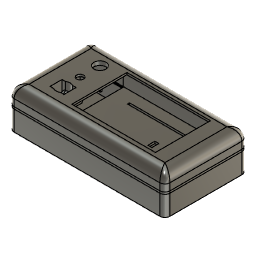
Case (Autodesk Fusion 360 design; units mm, degrees)
Autodesk Fusion 360 part; units mm, degrees
sketch "Base" plane through (0, 0, 0) normal (0, 0, 1) x (1, 0, 0)
  line L0 (1.2621, 68) -> (1.2621, 5)
  line L1 (1.2621, 5) -> (107, 5)
  line L2 (107, 5) -> (107, 68)
  line L3 (107, 68) -> (1.2621, 68)
  line L4 (-38.7379, 72.5) -> (-38.7379, 0.5)
  line L5 (-33.7379, -4.5) -> (112, -4.5)
  line L6 (117, 0.5) -> (117, 72.5)
  line L7 (112, 77.5) -> (-33.7379, 77.5)
  arc A0 (-33.7379, 77.5) -> (-38.7379, 72.5) centre (-33.7379, 72.5) ccw
  arc A1 (117, 72.5) -> (112, 77.5) centre (112, 72.5) ccw
  arc A2 (112, -4.5) -> (117, 0.5) centre (112, 0.5) ccw
  arc A3 (-38.7379, 0.5) -> (-33.7379, -4.5) centre (-33.7379, 0.5) ccw
  line L8 (39.1311, 77.5) -> (39.1311, -4.5)
  line L9 (-38.7379, 36.5) -> (117, 36.5)
  point P0 (-33.7379, 57.5)
  point P1 (-33.7379, 15.5)
  point P2 (112, 57.5)
  point P3 (112, 15.5)
  dimension "d4" = 9.5
  dimension "d5" = 10
  dimension "d7" = 5
  dimension "d8" = 40
  dimension "d72" = 9.5
  dimension "d73" = 63
  dimension "d74" = 105.7379
  dimension "d75" = 20
  dimension "d76" = 5
  constraint tangent L4 A0
  constraint tangent L7 A0
  constraint tangent L6 A1
  constraint tangent L7 A1
  constraint equal A0 A1
  constraint tangent L5 A2
  constraint tangent L6 A2
  constraint equal A0 A2
  constraint tangent L4 A3
  constraint tangent L5 A3
  constraint equal A0 A3
  constraint midpoint L7 L8.start
  constraint midpoint L5 L8.end
  constraint perpendicular L5 L8
  constraint midpoint L4 L9.start
  constraint midpoint L6 L9.end
  constraint symmetric L9 P0 P1
  constraint symmetric L8 P0 P2
  constraint symmetric L8 P1 P3
  measures "d4" distance of L1 L5
  measures "d5" distance of L2 L6
  measures "d7" radius of A0
  measures "d8" distance of L0 L4
  measures "d72" distance of L3 L7
  measures "d73" distance of L1 L3
  measures "d74" distance of L0 L2
  measures "d75" distance of L7 P0
  measures "d76" distance of L4 P0
extrude "Extrude1" add sketch "Base" along normal blind 20 makes body 1
sketch "Battery Inset" plane through (0, 0, 20) normal (0, 0, 1) x (-1, 0, 0)
  arc A0 (38.7379, -0.5) -> (33.7379, 4.5) centre (33.7379, -0.5) ccw
  line L0 (33.7379, 4.5) -> (-112, 4.5)
  arc A1 (-112, 4.5) -> (-117, -0.5) centre (-112, -0.5) ccw
  line L1 (-117, -0.5) -> (-117, -72.5)
  arc A2 (-117, -72.5) -> (-112, -77.5) centre (-112, -72.5) ccw
  line L2 (-112, -77.5) -> (33.7379, -77.5)
  arc A3 (33.7379, -77.5) -> (38.7379, -72.5) centre (33.7379, -72.5) ccw
  line L3 (38.7379, -72.5) -> (38.7379, -0.5)
  line L4 (-6.5, -68) -> (-107, -68)
  line L5 (-107, -68) -> (-107, -5)
  line L6 (-107, -5) -> (-6.5, -5)
  line L7 (-6.5, -5) -> (-6.5, -68)
  line L8 (-6.5, -36.5) -> (-107, -36.5) construction
  line L9 (38.7379, -36.5) -> (-117, -36.5) construction
  line L10 (28.7379, -68) -> (-107, -68)
  line L11 (-107, -68) -> (-107, -5)
  line L12 (-107, -5) -> (28.7379, -5)
  line L13 (28.7379, -5) -> (28.7379, -68)
  line L14 (-1.2621, -5) -> (-107, -5)
  line L15 (-107, -5) -> (-107, -68)
  line L16 (-107, -68) -> (-1.2621, -68)
  line L17 (38.7379, -72.5) -> (38.7379, -0.5)
  line L18 (-6.5, -68) -> (-3.5, -68)
  line L19 (-3.5, -68) -> (-3.5, -5)
  line L20 (-3.5, -5) -> (-6.5, -5)
  line L21 (-6.5, -5) -> (-6.5, -68)
  line L22 (-3.5, -12) -> (-6.5, -12)
  line L23 (-3.5, -30) -> (-6.5, -30)
  line L24 (-18.5, -44) -> (-22.5, -44)
  line L25 (-22.5, -44) -> (-22.5, -29)
  line L26 (-22.5, -29) -> (-18.5, -29)
  line L27 (-18.5, -29) -> (-18.5, -44)
  line L28 (-18.5, -36.5) -> (-22.5, -36.5) construction
  line L29 (-20.5, -44) -> (-20.5, -29) construction
  dimension "d168" = 63
  dimension "d169" = 100.5
  dimension "d170" = 10
  dimension "d171" = 3
  dimension "d174" = 15
  dimension "d175" = 4
  dimension "d176" = 14
  dimension "d188" = 7
  dimension "d189" = 25
  constraint horizontal L4
  constraint vertical L5
  constraint horizontal L6
  constraint vertical L7
  constraint midpoint L7 L8.start
  constraint midpoint L5 L8.end
  constraint collinear L8 L9
  constraint horizontal L10
  constraint vertical L11
  constraint horizontal L12
  constraint vertical L13
  constraint collinear L12 L14
  constraint collinear L11 L15
  constraint collinear L10 L16
  constraint horizontal L18
  constraint vertical L19
  constraint horizontal L20
  constraint vertical L21
  constraint collinear L6 L20
  constraint coincident L19 L22.start
  constraint coincident L7 L22.end
  constraint perpendicular L7 L22
  constraint coincident L19 L23.start
  constraint coincident L7 L23.end
  constraint perpendicular L7 L23
  constraint horizontal L24
  constraint vertical L25
  constraint horizontal L26
  constraint vertical L27
  constraint midpoint L27 L28.start
  constraint midpoint L25 L28.end
  constraint collinear L8 L28
  constraint midpoint L24 L29.start
  constraint midpoint L26 L29.end
  constraint collinear L5 L11
  measures "d168" distance of L4 L6
  measures "d169" distance of L5 L7
  measures "d170" distance of L13 L17
  measures "d171" distance of L7 L19
  measures "d174" distance of L24 L26
  measures "d175" distance of L25 L27
  measures "d176" distance of L7 L29
  measures "d188" distance of L20 L22
  measures "d189" distance of L20 L23
extrude "Extrude2" cut sketch "Battery Inset" against normal blind 17 contours L4 L5 L6 L7 L10 L11 L12 L14 L15 L16 L21 | L7 L19 L21 L22 L23 | L10 L12 L13 L14 L16 L19 | L24 L25 L26 L27 bodies 1
extrude "Extrude17" cut sketch "Battery Inset" against normal through all contours L24 L25 L26 L27 bodies 1
fillet "Fillet3" radius 0.5 12 edges at (56.75, 68, 20) (107, 36.5, 20) (56.75, 5, 20) (6.5, 49, 20) (5, 30, 20) (3.5, 49, 20) (-12.6189, 68, 20) (-28.7379, 36.5, 20) (-12.6189, 5, 20) (3.5, 8.5, 20) (6.5, 8.5, 20) (5, 12, 20) on bodies 1
sketch "Top Base" plane through (0, 0, 20) normal (0, 0, 1) x (-1, 0, 0)
  arc A0 (38.7379, -0.5) -> (33.7379, 4.5) centre (33.7379, -0.5) ccw
  line L0 (33.7379, 4.5) -> (-112, 4.5)
  arc A1 (-112, 4.5) -> (-117, -0.5) centre (-112, -0.5) ccw
  line L1 (-117, -0.5) -> (-117, -72.5)
  arc A2 (-117, -72.5) -> (-112, -77.5) centre (-112, -72.5) ccw
  line L2 (-112, -77.5) -> (33.7379, -77.5)
  arc A3 (33.7379, -77.5) -> (38.7379, -72.5) centre (33.7379, -72.5) ccw
  line L3 (38.7379, -72.5) -> (38.7379, -0.5)
  line L4 (29.2379, -68.5) -> (-4, -68.5)
  line L5 (-4, -68.5) -> (-4, -4.5)
  line L6 (-4, -4.5) -> (29.2379, -4.5)
  line L7 (29.2379, -4.5) -> (29.2379, -68.5)
  line L8 (-100.5103, -56.4999) -> (-100.5103, -10.4999)
  line L9 (-96.5103, -6.4999) -> (-20.5103, -6.4999)
  line L10 (-20.5103, -54.4999) -> (-92.5415, -54.4999)
  line L11 (-96.5103, -54.4999) -> (-96.5103, -10.4999)
  line L12 (-96.5103, -8.4999) -> (-20.5103, -8.4999)
  line L13 (-66.5103, -35.9999) -> (-70.5103, -35.9999)
  line L14 (-70.5103, -35.9999) -> (-70.5103, -28.9999)
  line L15 (-70.5103, -28.9999) -> (-66.5103, -28.9999)
  line L16 (-66.5103, -28.9999) -> (-66.5103, -35.9999)
  circle A4 centre (-8.5103, -14.4999) radius 5
  line L17 (-20.5103, -6.4999) -> (-20.5103, -8.4999)
  line L18 (-20.5103, -54.4999) -> (-20.5103, -56.4999)
  line L19 (-96.5103, -6.4999) -> (-96.5103, -8.4999)
  line L20 (-96.5103, -10.4999) -> (-100.5103, -10.4999)
  line L21 (-92.5415, -54.4999) -> (-92.5415, -56.4999)
  line L22 (-96.5103, -56.4999) -> (-96.5103, -54.4999)
  line L23 (-20.5103, -56.4999) -> (-92.5415, -56.4999)
  line L24 (-96.5103, -56.4999) -> (-100.5103, -56.4999)
  line L25 (-6, -4.5) -> (-6, -11.5)
  line L26 (-6, -11.5) -> (-4, -11.5)
  line L27 (-4, -11.5) -> (-4, -4.5)
  line L28 (-4, -4.5) -> (29.2379, -4.5)
  line L29 (29.2379, -4.5) -> (29.2379, -68.5)
  line L30 (29.2379, -68.5) -> (-4, -68.5)
  line L31 (-4, -68.5) -> (-4, -30.5)
  line L32 (-4, -30.5) -> (-6, -30.5)
  line L33 (-6, -30.5) -> (-6, -68.5)
  line L34 (-6, -68.5) -> (-107.5, -68.5)
  line L35 (-107.5, -68.5) -> (-107.5, -4.5)
  line L36 (-107.5, -4.5) -> (-6, -4.5)
  dimension "d32" = 50
  dimension "d33" = 2
  dimension "d34" = 2
  dimension "d35" = 4
  dimension "d36" = 80
  dimension "d37" = 34
  dimension "d38" = 4
  dimension "d39" = 7
  dimension "d40" = 29.5
  dimension "d41" = 10
  dimension "d42" = 92
  dimension "d43" = 8
  constraint horizontal L4
  constraint vertical L5
  constraint horizontal L6
  constraint vertical L7
  constraint horizontal L23
  constraint vertical L8
  constraint horizontal L9
  constraint vertical L17
  constraint horizontal L10
  constraint vertical L11
  constraint horizontal L12
  constraint horizontal L13
  constraint vertical L14
  constraint horizontal L15
  constraint vertical L16
  constraint collinear L17 L18
  constraint vertical L19
  constraint horizontal L20
  constraint vertical L21
  constraint vertical L22
  constraint collinear L23 L24
  constraint collinear L7 L29
  constraint collinear L4 L30
  constraint collinear L6 L28
  constraint collinear L5 L27
  measures "d32" distance of L9 L23
  measures "d33" distance of L10 L23
  measures "d34" distance of L9 L12
  measures "d35" distance of L8 L11
  measures "d36" distance of L8 L17
  measures "d37" distance of L8 L16
  measures "d38" distance of L14 L16
  measures "d39" distance of L13 L15
  measures "d40" distance of L9 L13
  measures "d41" diameter of A4
  measures "d42" distance of L8 A4.centre
  measures "d43" distance of L9 A4.centre
extrude "Extrude5" add sketch "Top Base" along normal blind 2 separate body contours A0 L0 A1 L1 A2 L2 A3 L3 | L5 A4 L25 L32 L33 L34 L35 L36 | L5 A4 L26 makes body 2
sketch "Top" plane through (0, 0, 22) normal (0, 0, 1) x (-1, 0, 0)
  line L0 (38.7379, -72.5) -> (38.7379, -0.5)
  arc A0 (38.7379, -0.5) -> (33.7379, 4.5) centre (33.7379, -0.5) ccw
  line L1 (33.7379, 4.5) -> (-112, 4.5)
  arc A1 (-112, 4.5) -> (-117, -0.5) centre (-112, -0.5) ccw
  line L2 (-117, -0.5) -> (-117, -72.5)
  arc A2 (-117, -72.5) -> (-112, -77.5) centre (-112, -72.5) ccw
  line L3 (-112, -77.5) -> (33.7379, -77.5)
  arc A3 (33.7379, -77.5) -> (38.7379, -72.5) centre (33.7379, -72.5) ccw
  line L4 (-3.4004, -67.4999) -> (-105.5103, -67.4999)
  line L5 (-105.5103, -67.4999) -> (-105.5103, -4.4999)
  line L6 (-105.5103, -4.4999) -> (-3.4004, -4.4999)
  line L7 (-3.4004, -4.4999) -> (-3.4004, -67.4999)
  line L8 (28.7379, -67.5) -> (-3.4004, -67.5)
  line L9 (-3.4004, -67.5) -> (-3.4004, -5.5)
  line L10 (-3.4004, -5.5) -> (28.7379, -5.5)
  line L11 (28.7379, -5.5) -> (28.7379, -67.5)
  line L12 (-96.5103, -8.4999) -> (-96.5103, -6.4999)
  line L13 (-100.5103, -10.4999) -> (-96.5103, -10.4999)
  line L14 (-20.5103, -56.4999) -> (-92.5415, -56.4999)
  line L15 (-92.5415, -56.4999) -> (-92.5415, -54.4999)
  line L16 (-96.5103, -8.4999) -> (-20.5103, -8.4999)
  line L17 (-96.5103, -54.4999) -> (-96.5103, -10.4999)
  line L18 (-4, -68.5) -> (-4, -16.658)
  line L19 (-93.5103, -67.4999) -> (-93.5103, -4.4999)
  dimension "d54" = 10
  dimension "d55" = 10
  dimension "d56" = 10
  dimension "d77" = 4
  dimension "d78" = 9
  dimension "d192" = 12
  constraint horizontal L4
  constraint vertical L5
  constraint horizontal L6
  constraint vertical L7
  constraint horizontal L8
  constraint vertical L9
  constraint horizontal L10
  constraint vertical L11
  constraint collinear L7 L9
  constraint coincident L4 L19.start
  constraint coincident L6 L19.end
  constraint perpendicular L6 L19
  measures "d54" distance of L3 L8
  measures "d55" distance of L1 L10
  measures "d56" distance of L0 L11
  measures "d77" distance of L6 L16
  measures "d78" distance of L5 L17
  measures "d192" distance of L5 L19
extrude "Extrude6" add sketch "Top" along normal blind 17 separate body contours L0 A0 L1 A1 L2 A2 L3 A3 | L4 L6 L7 L9 L19 | L4 L5 L6 L19 | L7 L8 L9 L10 L11 makes body 3
extrude "Extrude7" cut sketch "Top" along normal blind 15 contours L4 L6 L7 L9 L19 | L4 L5 L6 L19 bodies 3
extrude "Extrude8" cut sketch "Top" along normal blind 13 contours L7 L8 L9 L10 L11 bodies 3
extrude "Extrude19" cut sketch "Top" along normal blind 15.5 contours L4 L5 L6 L19 bodies 3
sketch "Screen Cutout" plane through (0, 0, 39) normal (0, 0, 1) x (-1, 0, 0)
  arc A0 (33.7379, -77.5) -> (38.7379, -72.5) centre (33.7379, -72.5) ccw
  line L0 (38.7379, -72.5) -> (38.7379, -0.5)
  arc A1 (38.7379, -0.5) -> (33.7379, 4.5) centre (33.7379, -0.5) ccw
  line L1 (33.7379, 4.5) -> (-112, 4.5)
  arc A2 (-112, 4.5) -> (-117, -0.5) centre (-112, -0.5) ccw
  line L2 (-117, -0.5) -> (-117, -72.5)
  arc A3 (-117, -72.5) -> (-112, -77.5) centre (-112, -72.5) ccw
  line L3 (-112, -77.5) -> (33.7379, -77.5)
  line L4 (-10.0103, -64.4999) -> (-93.5103, -64.4999)
  line L5 (-93.5103, -64.4999) -> (-93.5103, -9.4999)
  line L6 (-93.5103, -9.4999) -> (-10.0103, -9.4999)
  line L7 (-10.0103, -9.4999) -> (-10.0103, -64.4999)
  dimension "d59" = 83.5
  dimension "d60" = 55
  constraint horizontal L4
  constraint vertical L5
  constraint horizontal L6
  constraint vertical L7
  measures "d59" distance of L5 L7
  measures "d60" distance of L4 L6
extrude "Extrude9" cut sketch "Screen Cutout" against normal through all contours L4 L5 L6 L7 bodies 3
fillet "Fillet4" radius 10 8 edges at (117, 36.5, 39) (115.5355, 76.0355, 39) (39.1311, 77.5, 39) (-37.2734, 76.0355, 39) (-38.7379, 36.5, 39) (-37.2734, -3.0355, 39) (39.1311, -4.5, 39) (115.5355, -3.0355, 39) on bodies 3
hole "Hole2" at (-33.7379, 15.5, 0) at (-33.7379, 57.5, 0) at (112, 15.5, 0) at (112, 57.5, 0) direction (0, 0, 1) diameter 3.5 depth 30 tip angle 180 countersink diameter 7 countersink angle 90 bodies 1 2 3
ref_plane "WorkPlane1" through (39.1311, 36.5, 24) normal (0, 0, -1) x (1, 0, 0)
sketch "Insets" plane through (39.1311, 36, 24) normal (0, 0, -1) x (1, 0, 0)
  line L0 (77.8689, 35.5) -> (77.8689, -36.5)
  line L1 (67.8689, 31) -> (67.8689, -32)
  line L2 (-77.8689, -0.5) -> (77.8689, -0.5)
  line L3 (66.3792, -31.4999) -> (66.3792, 31.5001)
  line L4 (-77.8689, -36.5) -> (-77.8689, 35.5)
  line L5 (-67.8689, 30.5) -> (-67.8689, -31.5)
  line L6 (72.8689, -41.5) -> (-72.8689, -41.5)
  circle A0 centre (-72.8689, -21.5) radius 2.3
  circle A1 centre (72.8689, -21.5) radius 2.3
  circle A2 centre (-72.8689, 20.5) radius 2.3
  circle A3 centre (72.8689, 20.5) radius 2.3
  point P0 (-72.8689, -21.5)
  point P1 (72.8689, -21.5)
  point P2 (-72.8689, 21)
  point P3 (72.8689, 21)
  dimension "d193" = 4.6
  constraint coincident P0 A0.centre
  constraint coincident P1 A1.centre
  constraint equal A0 A1
  constraint symmetric L2 A0 A2
  constraint symmetric L2 A1 A3
  measures "d193" diameter of A0
extrude "Thread inserts cut" cut sketch "Insets" against normal blind 7.5 from surface at 2 bodies 3
chamfer "Chamfer6" distance 1 angle 45 4 edges at (109.8556, 56.6683, 22) (109.8556, 14.6683, 22) (-35.8823, 14.6683, 22) (-35.8823, 56.6683, 22) on bodies 3
sketch "Buttons" plane through (0, 0, 39) normal (0, 0, 1) x (-1, 0, 0)
  line L0 (-10.0103, -9.4999) -> (-10.0103, -64.4999)
  line L1 (-10.0103, -64.4999) -> (-93.5103, -64.4999)
  line L2 (-93.5103, -64.4999) -> (-93.5103, -9.4999)
  line L3 (-93.5103, -9.4999) -> (-10.0103, -9.4999)
  line L4 (-107, -5.5) -> (-107, -67.5)
  line L5 (-107, -67.5) -> (28.7379, -67.5)
  line L6 (28.7379, -67.5) -> (28.7379, -5.5)
  line L7 (28.7379, -5.5) -> (-107, -5.5)
  circle A0 centre (9.3638, -56.9428) radius 6
  circle A1 centre (9.3638, -37.1549) radius 3.5
  line L8 (18.3638, -28.1549) -> (18.3638, -46.1549)
  line L9 (18.3638, -46.1549) -> (-3.6362, -46.1549)
  line L10 (-3.6362, -46.1549) -> (-3.6362, -28.1549)
  line L11 (-3.6362, -28.1549) -> (18.3638, -28.1549)
  line L12 (19.25, -47.7455) -> (-1.9181, -47.7455)
  line L13 (-1.9181, -47.7455) -> (-1.9181, -12.0036)
  line L14 (-1.9181, -12.0036) -> (19.25, -12.0036)
  line L15 (19.25, -12.0036) -> (19.25, -47.7455)
  line L16 (16.3638, -26.0524) -> (2.3638, -26.0524)
  line L17 (2.3638, -26.0524) -> (2.3638, -14.0524)
  line L18 (2.3638, -14.0524) -> (16.3638, -14.0524)
  line L19 (16.3638, -14.0524) -> (16.3638, -26.0524)
  line L20 (9.3638, -26.0524) -> (9.3638, -14.0524) construction
  line L21 (16.3638, -20.0524) -> (2.3638, -20.0524) construction
  circle A2 centre (9.3638, -20.0524) radius 7
  line L22 (-10.0103, -64.4999) -> (28.7379, -64.4999) construction
  line L23 (9.3638, -64.4999) -> (9.3638, -5.5) construction
  line L24 (14.3638, -26.0524) -> (14.3638, -14.0524)
  line L25 (4.3638, -26.0524) -> (4.3638, -14.0524)
  line L26 (10.6138, -29.6049) -> (8.1138, -29.6049)
  line L27 (8.1138, -29.6049) -> (8.1138, -28.4049)
  line L28 (8.1138, -28.4049) -> (10.6138, -28.4049)
  line L29 (10.6138, -28.4049) -> (10.6138, -29.6049)
  line L30 (9.3638, -29.6049) -> (9.3638, -28.4049)
  circle A3 centre (9.3638, -37.1549) radius 6
  dimension "d122" = 12
  dimension "d124" = 7
  dimension "d125" = 18
  dimension "d126" = 22
  dimension "d127" = 9
  dimension "d128" = 9
  dimension "d145" = 14
  dimension "d146" = 12
  dimension "d147" = 14
  dimension "d152" = 2
  dimension "d153" = 2
  dimension "d198" = 2.5
  dimension "d199" = 1.2
  dimension "d200" = 8.75
  dimension "d204" = 12
  constraint horizontal L12
  constraint vertical L13
  constraint horizontal L14
  constraint vertical L15
  constraint horizontal L16
  constraint vertical L17
  constraint horizontal L18
  constraint vertical L19
  constraint midpoint L16 L20.start
  constraint midpoint L18 L20.end
  constraint midpoint L19 L21.start
  constraint midpoint L17 L21.end
  constraint midpoint L21 A2.centre
  constraint coincident L0.end L1.start
  constraint coincident L6 L22.end
  constraint perpendicular L6 L22
  constraint midpoint L22 L23.start
  constraint coincident L7 L23.end
  constraint perpendicular L7 L23
  constraint coincident A0.centre L23
  constraint coincident A2.centre L23
  constraint coincident A1.centre L23
  constraint coincident L16 L24.start
  constraint coincident L18 L24.end
  constraint perpendicular L18 L24
  constraint coincident L16 L25.start
  constraint coincident L18 L25.end
  constraint perpendicular L18 L25
  constraint horizontal L26
  constraint vertical L27
  constraint horizontal L28
  constraint vertical L29
  constraint midpoint L26 L30.start
  constraint midpoint L28 L30.end
  constraint collinear L23 L30
  constraint concentric A1 A3
  measures "d122" diameter of A0
  measures "d124" diameter of A1
  measures "d125" distance of L8.start L8.end
  measures "d126" distance of L8 L10
  measures "d127" distance of A1.centre L11
  measures "d128" distance of A1.centre L8
  measures "d145" distance of L17 L19
  measures "d146" distance of L16 L18
  measures "d147" diameter of A2
  measures "d152" distance of L17 L25
  measures "d153" distance of L19 L24
  measures "d198" distance of L26.start L26.end
  measures "d199" distance of L26.start L28.end
  measures "d200" distance of A1.centre L28
  measures "d204" diameter of A3
extrude "Extrude13" add sketch "Buttons" against normal blind 12 contours L8 L9 L11 L12 L13 L14 L15 | L16 L19 A2 L24 | L16 A2 L24 | L18 L19 A2 L24 | A2 L24 | L16 A2 | L16 L18 A2 L24 L25 | L18 A2 L24 | L16 A2 L25 | L18 A2 | L16 L17 A2 L25 | A2 L25 | L18 A2 L25 | L17 L18 A2 L25 bodies 3
extrude "Extrude11" cut sketch "Buttons" against normal through all contours A0 | A1 bodies 3
extrude "Extrude15" cut sketch "Buttons" against normal through all contours L16 L19 A2 L24 | L18 L19 A2 L24 | A2 L24 | L16 L17 A2 L25 | A2 L25 | L17 L18 A2 L25 bodies 3
extrude "Extrude16" cut sketch "Buttons" against normal blind 10 contours L16 A2 L24 | A2 L24 | L16 A2 | L16 L18 A2 L24 L25 | L18 A2 L24 | L16 A2 L25 | L18 A2 | A2 L25 | L18 A2 L25 bodies 3
extrude "Extrude21" cut sketch "Buttons" along normal blind 3 from surface at -4 contours L26 L28 L29 L30 | L26 L27 L28 L30 bodies 3
extrude "Extrude22" cut sketch "Buttons" along normal blind 2 from surface at -4 contours A3 bodies 3
chamfer "Chamfer5" distance 2 distance2 5.99 6 edges at (-13.6666, 26.0524, 29) (-9.3638, 27.0524, 29) (-5.061, 26.0524, 29) (-13.6666, 14.0524, 29) (-9.3638, 13.0524, 29) (-5.061, 14.0524, 29) measured on face at (-14.5657, 26.0524, 35.6667) measured on face at (-6.0324, 26.2089, 35.6667) measured on face at (-4.162, 26.0524, 35.6667) measured on face at (-14.5657, 14.0524, 35.6667) measured on face at (-9.6794, 13.0595, 32.3333) measured on face at (-4.162, 14.0524, 35.6667) on bodies 3
sketch "Inspection Sketch" plane through (0, 0, 22) normal (0, 0, -1) x (1, 0, 0)
  line L0 (-28.7379, -5.5) -> (3.4004, -5.5)
  line L1 (3.4004, -5.5) -> (3.4004, -4.4999)
  line L2 (3.4004, -4.4999) -> (105.5103, -4.4999)
  line L3 (105.5103, -4.4999) -> (105.5103, -67.4999)
  line L4 (105.5103, -67.4999) -> (3.4004, -67.4999)
  line L5 (3.4004, -67.5) -> (-28.7379, -67.5)
  line L6 (-28.7379, -67.5) -> (-28.7379, -5.5)
  arc A0 (-38.7379, -72.5) -> (-33.7379, -77.5) centre (-33.7379, -72.5) ccw
  line L7 (-33.7379, -77.5) -> (112, -77.5)
  arc A1 (112, -77.5) -> (117, -72.5) centre (112, -72.5) ccw
  line L8 (117, -72.5) -> (117, -0.5)
  arc A2 (117, -0.5) -> (112, 4.5) centre (112, -0.5) ccw
  line L9 (112, 4.5) -> (-33.7379, 4.5)
  arc A3 (-33.7379, 4.5) -> (-38.7379, -0.5) centre (-33.7379, -0.5) ccw
  line L10 (-38.7379, -0.5) -> (-38.7379, -72.5)
  line L11 (-19.25, -12.0036) -> (-19.25, -47.7455)
  line L12 (-19.25, -47.7455) -> (1.9181, -47.7455)
  line L13 (1.9181, -47.7455) -> (1.9181, -46.1549)
  line L14 (1.9181, -46.1549) -> (1.9181, -47.7455)
  line L15 (1.9181, -47.7455) -> (-19.25, -47.7455)
  line L16 (-19.25, -47.7455) -> (-19.25, -12.0036)
  line L17 (3.4004, -5.5) -> (-28.7379, -5.5)
  line L18 (-28.7379, -5.5) -> (-28.7379, -67.5)
  line L19 (-28.7379, -67.5) -> (3.4004, -67.5)
  line L20 (3.4004, -67.4999) -> (3.4004, -5.5)
  line L21 (-14.3638, -14.0524) -> (-14.3638, -26.0524)
  line L22 (-14.3638, -26.0524) -> (-16.3638, -26.0524)
  line L23 (-16.3638, -26.0524) -> (-16.3638, -14.0524)
  line L24 (-16.3638, -14.0524) -> (-14.3638, -14.0524)
  line L25 (-2.3638, -14.0524) -> (-2.3638, -26.0524)
  line L26 (-2.3638, -26.0524) -> (-4.3638, -26.0524)
  line L27 (-4.3638, -26.0524) -> (-4.3638, -14.0524)
  line L28 (-4.3638, -14.0524) -> (-2.3638, -14.0524)
  line L29 (-18.3638, -46.1549) -> (-18.3638, -28.1549)
  line L30 (-18.3638, -28.1549) -> (1.9181, -28.1549)
  line L31 (1.9181, -28.1549) -> (1.9181, -12.0036)
  line L32 (1.9181, -12.0036) -> (-19.25, -12.0036)
  line L33 (-19.25, -12.0036) -> (1.9181, -12.0036)
  line L34 (1.9181, -12.0036) -> (1.9181, -28.1549)
  circle A4 centre (-9.3638, -56.9428) radius 6
  circle A5 centre (-33.7379, -15.5) radius 3.3
  circle A6 centre (112, -57.5) radius 3.3
  circle A7 centre (112, -15.5) radius 3.3
  circle A8 centre (-33.7379, -57.5) radius 3.3
  line L35 (1.9181, -46.1549) -> (-18.3638, -46.1549)
  circle A9 centre (-9.3638, -37.1549) radius 6
  line L36 (-10.6138, -28.4049) -> (-8.1138, -28.4049)
  line L37 (-8.1138, -28.4049) -> (-8.1138, -29.6049)
  line L38 (-8.1138, -29.6049) -> (-10.6138, -29.6049)
  line L39 (-10.6138, -29.6049) -> (-10.6138, -28.4049)
  line L40 (-18.3638, -28.1549) -> (-18.3638, -46.1549)
  line L41 (-18.3638, -46.1549) -> (1.9181, -46.1549)
  line L42 (1.9181, -28.1549) -> (-18.3638, -28.1549)
  line L43 (3.4004, -67.4999) -> (3.4004, -67.5)
  line L44 (3.4004, -67.5) -> (3.4004, -67.4999)
  dimension "d157" = 9.4879
  dimension "d164" = 19.7544
  measures "d157" distance of L11 L18
  measures "d164" distance of L4 L15
equation "d9 = 15 mm + 5 mm"
named bodies: "Base", "Middle", "Top"
